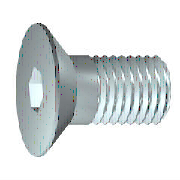
# Autodesk Inventor part: DIN 7991 - M5x8
Saved by Autodesk Inventor 2022.2 (Build 262287000, 287)
## iProperties
Created: 2021-02-02
Part Number: DIN 7991 - M5x8
Material: Stahl, weich
Description: Senkschrauben mit Innensechskant
Document SubType Name: Modeling
Standard: DIN 7991
Designer: jan
Standards Organization: DIN
Language: de-DE
Size Designation: M5x8
Categories: <MemberInstance><Categories><Category DisplayName="Verbindungselemente" InternalName="e4da775c-781d-43d5-af7c-5136215cf5a6" Mnemonic="FSTN"><Category DisplayName="Schrauben" InternalName="536e6df0-f778-49ac-b2f2-25c71d2aa0b2" Mnemonic="SCRW"><CategoryParameter DisplayName="Bezeichnung des Nenndurchmessers" InternalName="03caf894-eafd-4c09-a035-916ac084b87b" Mnemonic="nomdiadesig"/><CategoryParameter DisplayName="Nennlänge" InternalName="238ecbaf-3e6c-45dd-aa95-4068c8e0fd02" Mnemonic="nomlen"/><CategoryParameter DisplayName="Gewindebezeichnung" InternalName="586d5e89-370a-4089-914f-0110033585c7" Mnemonic="thrdesign"/><CategoryParameter DisplayName="Gewindeserienbeschreibung" InternalName="87c5849c-b3a5-4c3e-9c9b-2feecef9be86" Mnemonic="thrserdsgn"/><CategoryParameter DisplayName="Nenndurchmesser" InternalName="8bbe3f8e-44cf-40a9-a251-3a6edc8168d6" Mnemonic="nomdia"/><CategoryParameter DisplayName="Gewindeart" InternalName="b4bbb7bc-d6aa-4c9f-a9a9-4152b9f6fe49" Mnemonic="thrtype"/><CategoryParameter DisplayName="Gewindesteigung" InternalName="bb82302e-82d8-4176-8fc1-c5d7bb17d5ad" Mnemonic="pitch1"/><CategoryParameter DisplayName="Windungen pro Einheit" InternalName="bdc6e7d2-ffd0-4d9c-a173-16b95ebb912d" Mnemonic="thrperunit1"/><CategoryParameter DisplayName="Gewindeklasse" InternalName="ebc0d23b-2cc6-4d2a-b376-d52aae53bab6" Mnemonic="thrclss"/><Category DisplayName="Senkkopf" InternalName="49656530-5684-4604-a233-68d537625f23" Mnemonic="CSSCRW"><CategoryParameter DisplayName="Typ" InternalName="161b33bb-bee3-4fab-a17d-97511dff40f0" Mnemonic="type"/><CategoryParameter DisplayName="Gewindelänge" InternalName="207f0278-6dec-43ab-bffc-1c6d03e64de4" Mnemonic="thrlen"/><CategoryParameter DisplayName="Grifflänge" InternalName="2fff3de5-ce2a-45fd-9425-99ddc9dff352" Mnemonic="grplen"/><CategoryParameter DisplayName="Eigenschaftenklasse" InternalName="5249b721-5ecc-4781-a2e8-d7e3bda3ecca" Mnemonic="propclss"/><CategoryParameter DisplayName="Kopfhöhe" InternalName="57526df9-da71-45fb-acb4-1d0529a34778" Mnemonic="headh"/><CategoryParameter DisplayName="Schaftdurchmesser" InternalName="7ece923f-d8ee-40d5-83f8-980cad520964" Mnemonic="grpdia"/><CategoryParameter DisplayName="Kopfdurchmesser" InternalName="a509cd31-06d1-44c5-b54e-d7a695352906" Mnemonic="headdia"/><CategoryParameter DisplayName="Kopfwinkel" InternalName="dbcfc1e0-7990-403e-bc2e-90d1c639222a" Mnemonic="headang"/></Category></Category></Category><Category DisplayName="Datentyp" InternalName="23b78d0f-2648-40c6-8793-ca6db495c9e8" Mnemonic="DATATYPE"><CategoryParameter DisplayName="Anzeigename" InternalName="05415f3d-3907-474b-a020-eb9d644f4cf3" Mnemonic="DISPLAYNAME"/><CategoryParameter DisplayName="Norm" InternalName="0c0a119c-1e12-4c84-803f-101930972f5e" Mnemonic="STANDARD"/><CategoryParameter DisplayName="Beschreibung" InternalName="13903e3d-64b1-4950-80da-f627842ea37f" Mnemonic="DESCRIPTION"/><CategoryParameter DisplayName="Bezeichnung" InternalName="2675968c-4ce5-49e0-a4f5-552d29089031" Mnemonic="DESIGNATION"/><CategoryParameter DisplayName="Standardzeile" InternalName="2af9ec52-faaa-4026-b378-f9fa4afca842" Mnemonic="DEFAULTROW"/><CategoryParameter DisplayName="Ordnername" InternalName="3f06958e-8713-4116-9be7-ed6184ecc97b" Mnemonic="FOLDERNAME"/><CategoryParameter DisplayName="Revisionsanleitung" InternalName="45a75005-10b1-4dfc-8d6d-dfe629f0b93c" Mnemonic="REVISIONGUID"/><CategoryParameter DisplayName="Dateiname" InternalName="8b46a4cc-9585-4fed-90c3-899f57e09a73" Mnemonic="FILENAME"/><CategoryParameter DisplayName="Normungsorganisation" InternalName="8f5914e1-4693-403f-8ab5-d37768198c9d" Mnemonic="STDSORG"/><CategoryParameter DisplayName="Gruppenversion" InternalName="914462f6-6e19-4b14-ba84-155b9680b1d0" Mnemonic="FAMILYREVISION"/><CategoryParameter DisplayName="Normrevision" InternalName="91d5a463-65c2-4fde-b823-3b7fea5e8e17" Mnemonic="STANDARDREVISION"/><CategoryParameter DisplayName="Variantenrevision" InternalName="a65d44b9-392f-4f4f-857b-e4b3d54996fe" Mnemonic="MEMBERREVISION"/><CategoryParameter DisplayName="ClipFormat" InternalName="bc51e27b-3422-4e78-93ef-cec197ddf230" Mnemonic="CLIPFORMAT"/><CategoryParameter DisplayName="Hersteller" InternalName="cd6c7a72-a28a-4e50-99a9-2c7f4e13e5ad" Mnemonic="MANUFACTURER"/><CategoryParameter DisplayName="InternerName" InternalName="cf1d0246-76d9-4b4a-8305-fa0409afb5c1" Mnemonic="INTERNALNAME"/><CategoryParameter DisplayName="IstMetrisch" InternalName="e2385c5b-1ea4-4823-96a8-8de651266ec3" Mnemonic="ISMETRIC"/><Category DisplayName="Bauteil" InternalName="c0e0b642-3bcb-4cc8-9e80-f96d35c4afa4" Mnemonic="PART"><CategoryParameter DisplayName="Bauteilnummer" InternalName="016b6077-bfbe-49bd-92c9-d8d59c39c941" Mnemonic="PARTNUMBER"/><CategoryParameter DisplayName="Bestandsnummer" InternalName="4dba7c1c-e26c-444e-836c-b08b433409a8" Mnemonic="STOCKNUMBER"/><CategoryParameter DisplayName="Materialschlüssel" InternalName="5c9a8adb-dd2b-4535-b97f-0a94a95fe41f" Mnemonic="MATERIALKEY"/><CategoryParameter DisplayName="Material" InternalName="818a152a-d3c3-49ca-80ee-df7d91421b8e" Mnemonic="MATERIAL"/></Category></Category><Category DisplayName="Abwärtskompatibilitätszuordnung DA" InternalName="924fff40-ddd0-4eff-ad42-30e3774ef79e" Mnemonic="LEGACYMAPDA"><CategoryParameter DisplayName="DA-Cookie" InternalName="316934ee-8fe1-4c7a-9c36-f2d79e1add1a" Mnemonic="DACOOKIE"/></Category></Categories><FamilyTemplate Id="D7991"><FamilyTemplateParameters><FamilyTemplateParameter ObjectType="kUserParameterObject" ValueType="xs:double" Id="1" ObjectReferenceKey="NND"/><FamilyTemplateParameter ObjectType="kUserParameterObject" ValueType="xs:double" Id="2" ObjectReferenceKey="NLG"/><FamilyTemplateParameter ObjectType="kUserParameterObject" ValueType="xs:double" Id="3" ObjectReferenceKey="PTC"/><FamilyTemplateParameter ObjectType="kUserParameterObject" ValueType="xs:double" Id="4" ObjectReferenceKey="dk"/><FamilyTemplateParameter ObjectType="kUserParameterObject" ValueType="xs:double" Id="5" ObjectReferenceKey="ParK"/><FamilyTemplateParameter ObjectType="kUserParameterObject" ValueType="xs:double" Id="6" ObjectReferenceKey="ParS"/><FamilyTemplateParameter ObjectType="kUserParameterObject" ValueType="xs:double" Id="7" ObjectReferenceKey="ParT"/><FamilyTemplateParameter ObjectType="kUserParameterObject" ValueType="xs:double" Id="8" ObjectReferenceKey="r"/><FamilyTemplateParameter ObjectType="kUserParameterObject" ValueType="xs:double" Id="9" ObjectReferenceKey="b"/><FamilyTemplateParameter ObjectType="kUserParameterObject" ValueType="xs:double" Id="10" ObjectReferenceKey="ParC"/><FamilyTemplateParameter ObjectType="kUserParameterObject" ValueType="xs:integer" Id="11" ObjectReferenceKey="ang"/><FamilyTemplateParameter ObjectType="kUserParameterObject" ValueType="xs:double" Id="120" ObjectReferenceKey="THREADDIA"/><FamilyTemplateParameter ObjectType="kPropertyObject" ValueType="xs:string" Id="100" ObjectReferenceKey="{32853F0F-3444-11d1-9E93-0060B03C1CA6}" SubObjectId="52"/><FamilyTemplateParameter ObjectType="kPropertyObject" ValueType="xs:string" Id="105" ObjectReferenceKey="{32853F0F-3444-11d1-9E93-0060B03C1CA6}" SubObjectId="5"/><FamilyTemplateParameter ObjectType="kPartComponentDefinitionObject" ValueType="xs:string" Id="110" SubObjectId="Material"/><FamilyTemplateParameter ObjectType="kThreadFeatureObject" ValueType="xs:structure" Id="300" ObjectReferenceKey="100200001000000033070000000000008000000000000000" SubObjectId="ThreadInfo"><FamilyTemplateParameter ObjectType="" ValueType="xs:string" Id="301" SubObjectId="ThreadDesignation"/><FamilyTemplateParameter ObjectType="" ValueType="xs:string" Id="302" SubObjectId="ThreadType"/><FamilyTemplateParameter ObjectType="" ValueType="xs:string" Id="303" SubObjectId="ThreadClass"/></FamilyTemplateParameter></FamilyTemplateParameters></FamilyTemplate><CategoryParameterMap><ParamToTemplateMap><ParamToTemplate CategoryParameter="//CategoryParameter[@InternalName='05415f3d-3907-474b-a020-eb9d644f4cf3']" ConstantValue="DIN 7991"/><ParamToTemplate CategoryParameter="//CategoryParameter[@InternalName='cf1d0246-76d9-4b4a-8305-fa0409afb5c1']" ConstantValue="DC008177-FB61-46D9-9B99-764838F13578"/><ParamToTemplate CategoryParameter="//CategoryParameter[@InternalName='3f06958e-8713-4116-9be7-ed6184ecc97b']" ConstantValue="DIN 7991(2)"/><ParamToTemplate CategoryParameter="//CategoryParameter[@InternalName='914462f6-6e19-4b14-ba84-155b9680b1d0']" ConstantValue="10"/><ParamToTemplate CategoryParameter="//CategoryParameter[@InternalName='bc51e27b-3422-4e78-93ef-cec197ddf230']" ConstantValue="CF_INVENTOR.STDPARTS"/><ParamToTemplate CategoryParameter="//CategoryParameter[@InternalName='e2385c5b-1ea4-4823-96a8-8de651266ec3']" ConstantValue="true"/><ParamToTemplate CategoryParameter="//CategoryParameter[@InternalName='13903e3d-64b1-4950-80da-f627842ea37f']" ConstantValue="Hexagon socket countersunk head cap screws"/><ParamToTemplate CategoryParameter="//CategoryParameter[@InternalName='8f5914e1-4693-403f-8ab5-d37768198c9d']" ConstantValue="DIN"/><ParamToTemplate CategoryParameter="//CategoryParameter[@InternalName='0c0a119c-1e12-4c84-803f-101930972f5e']" ConstantValue="DIN 7991"/><ParamToTemplate CategoryParameter="//CategoryParameter[@InternalName='cd6c7a72-a28a-4e50-99a9-2c7f4e13e5ad']" TemplateParameter="104"/><ParamToTemplate CategoryParameter="//CategoryParameter[@InternalName='91d5a463-65c2-4fde-b823-3b7fea5e8e17']" TemplateParameter="103"/><ParamToTemplate CategoryParameter="//CategoryParameter[@InternalName='45a75005-10b1-4dfc-8d6d-dfe629f0b93c']" ConstantValue="5cfd8028-8e28-42b2-9e56-1a0a1c172dc8"/><ParamToTemplate CategoryParameter="//CategoryParameter[@InternalName='2af9ec52-faaa-4026-b378-f9fa4afca842']" ConstantValue="10"/><ParamToTemplate CategoryParameter="//CategoryParameter[@InternalName='8b46a4cc-9585-4fed-90c3-899f57e09a73']" ConstantValue="DIN 7991 - M5x8"/><ParamToTemplate CategoryParameter="//CategoryParameter[@InternalName='a65d44b9-392f-4f4f-857b-e4b3d54996fe']" ConstantValue="B204BD3B-70D1-4571-AD84-C0F483FDBC28"/><ParamToTemplate CategoryParameter="//CategoryParameter[@InternalName='2fff3de5-ce2a-45fd-9425-99ddc9dff352']" ConstantValue="1,6"/><ParamToTemplate CategoryParameter="//CategoryParameter[@InternalName='03caf894-eafd-4c09-a035-916ac084b87b']" ConstantValue="M5"/><ParamToTemplate CategoryParameter="//CategoryParameter[@InternalName='316934ee-8fe1-4c7a-9c36-f2d79e1add1a']" ConstantValue="*DIN~D7991~M5x8~8*"/><ParamToTemplate CategoryParameter="//CategoryParameter[@InternalName='2675968c-4ce5-49e0-a4f5-552d29089031']" TemplateParameter="100"/><ParamToTemplate CategoryParameter="//CategoryParameter[@InternalName='818a152a-d3c3-49ca-80ee-df7d91421b8e']" TemplateParameter="110"/><ParamToTemplate CategoryParameter="//CategoryParameter[@InternalName='238ecbaf-3e6c-45dd-aa95-4068c8e0fd02']" TemplateParameter="2"/><ParamToTemplate CategoryParameter="//CategoryParameter[@InternalName='8bbe3f8e-44cf-40a9-a251-3a6edc8168d6']" TemplateParameter="1"/><ParamToTemplate CategoryParameter="//CategoryParameter[@InternalName='016b6077-bfbe-49bd-92c9-d8d59c39c941']" TemplateParameter="105"/><ParamToTemplate CategoryParameter="//CategoryParameter[@InternalName='bb82302e-82d8-4176-8fc1-c5d7bb17d5ad']" TemplateParameter="3"/><ParamToTemplate CategoryParameter="//CategoryParameter[@InternalName='57526df9-da71-45fb-acb4-1d0529a34778']" TemplateParameter="5"/><ParamToTemplate CategoryParameter="//CategoryParameter[@InternalName='ebc0d23b-2cc6-4d2a-b376-d52aae53bab6']" TemplateParameter="303"/><ParamToTemplate CategoryParameter="//CategoryParameter[@InternalName='586d5e89-370a-4089-914f-0110033585c7']" TemplateParameter="301"/><ParamToTemplate CategoryParameter="//CategoryParameter[@InternalName='b4bbb7bc-d6aa-4c9f-a9a9-4152b9f6fe49']" TemplateParameter="302"/><ParamToTemplate CategoryParameter="//CategoryParameter[@InternalName='dbcfc1e0-7990-403e-bc2e-90d1c639222a']" TemplateParameter="11"/><ParamToTemplate CategoryParameter="//CategoryParameter[@InternalName='207f0278-6dec-43ab-bffc-1c6d03e64de4']" TemplateParameter="9"/><ParamToTemplate CategoryParameter="//CategoryParameter[@InternalName='a509cd31-06d1-44c5-b54e-d7a695352906']" TemplateParameter="4"/></ParamToTemplateMap></CategoryParameterMap></MemberInstance>
Mass: 1.73562 g
Surface Area: 2.92468 cm^2
Volume: 0.221098 cm^3
Density: 7.85 g/cm^3
Appearance: Halbpoliert
IsCustomPart: 0
Author: jan
Autodesk Inventor part; units mm, degrees
ref_plane "YZ Plane" through (0, 0, 0) normal (1, 0, 0) x (0, 1, 0)
sketch "Skizze1" plane through (0, 0, 0) normal (0, 1, 0) x (-1, 0, 0)
  point P0 (0, 0)
sketch "Skizze2" plane through (0, 0, 0) normal (0, 1, 0) x (-1, 0, 0)
  line L0 (-2.5, -8) -> (0, -8)
  line L1 (-2.5, -2.8) -> (-2.5, -8)
  line L2 (-5, -0.3) -> (-2.5, -2.8)
  line L3 (-5, 0) -> (-5, -0.3)
  line L4 (0, 0) -> (-5, 0)
  line L5 (0, -8) -> (0, 0)
  line L6 (0, -8) -> (0, 0)
  line L7 (0, -9.6) -> (0, 1.6) projected
  line L8 (1, 0) -> (-6, 0) projected
  dimension "d3" = 5
  dimension "d5" = 2.5
  dimension "d7" = 8
  dimension "ParC" = 0.3
  dimension "d22" = 0
  dimension "d23" = 0
  dimension "d43" = 45
  constraints: 14 end point, 3 vertical, 2 horizontal
  measures "d3" distance of L4.start L3.start
  measures "d5" distance of L0.start L0.end
  measures "d7" distance of L0.end L4.start
  measures "ParC" distance of L3.start L2.start
  measures "d22" distance between parallel lines of L7 L5
  measures "d23" distance between parallel lines of L8 L4
  measures "d43" angle of L5 L2
revolve "Drehung1" add sketch "Skizze2" angle 360 about axis through (0, 0, -8) along (0, 0, -1)
sketch "Skizze3" plane through (0, 0, 0) normal (0, 0, 1) x (1, 0, 0)
  line L0 (-1.5, 0.866) -> (-1.5, -0.866)
  line L1 (0, 1.7321) -> (-1.5, 0.866)
  line L2 (1.5, 0.866) -> (0, 1.7321)
  line L3 (1.5, -0.866) -> (1.5, 0.866)
  line L4 (0, -1.7321) -> (1.5, -0.866)
  line L5 (-1.5, -0.866) -> (0, -1.7321)
  circle A0 centre (0, 0) radius 1.5 construction
  circle A1 centre (0, 0) radius 2.5 construction
  dimension "d11" = 3
  dimension "d13" = 120
  dimension "d15" = 120
  constraints: 12 end point, 6 tangent, 2 parallel, 2 vertical, 1 centre point, 1 concentric
  measures "d11" diameter of A0
  measures "d13" angle of L0 L1
  measures "d15" angle of L5 L0
extrude "Extrusion1" cut sketch "Skizze3" against normal blind 2.3
fillet "Rundung1" radius 0.2 1 edges at (-2.5, 0, -2.8)
chamfer "Fase1" distance 0.4 angle 45 1 edges at (-2.5, 0, -8) measured on face at (-0.599, -2.4272, -6.2943)
thread "Gewinde1" size "M5x0.8" class "6g" standard "ISO Metric profile" length 3.6
ref_plane "MSC_PF1" through (0, 0, 0) normal (1, 0, 0) x (0, 1, 0)
ref_plane "MSC_PT1" through (0, 0, 0) normal (0, 0, -1) x (-1, 0, 0)
equation "\"d3\" = 0.5 * dk"
equation "\"d5\" = 0.5 * NND"
equation "\"d7\" = NLG"
equation "\"d43\" = 0.5 * ang"
equation "\"d11\" = ParS"
equation "\"d16\" = ParT"
equation "\"d18\" = r"
equation "\"d19\" = 0.5 * PTC"
equation "\"d39\" = 0.5 * PTC"
equation "\"NND\" = 5"
equation "\"PTC\" = 0.8"
equation "\"ParK\" = 2.8"
equation "\"ParS\" = 3"
equation "\"ParT\" = 2.3"
equation "\"r\" = 0.2"
equation "\"NLG\" = 8"
equation "\"ang\" = 90deg"
equation "\"THREADDIA\" = NND"
equation "\"dk\" = 10"
body "Solid1"
